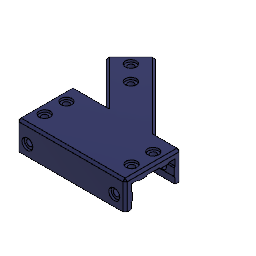
1-Side_Support_Top_Brace_Left v1 v1 (Autodesk Fusion 360 design; units mm, degrees)
Autodesk Fusion 360 part; units mm, degrees
mesh "Mesh1" [no effect]
sketch "Mesh Sectcion Sketch YZ" plane through (50, 0, 0) normal (1, 0, 0) x (0, 1, 0)
sketch "Sketch 2040" plane through (0, 0, 0) normal (1, 0, 0) x (0, 1, 0)
  line L0 (-4.607, 0) -> (-56.5, 0)
  line L1 (-56.5, 0.1599) -> (-56.5, 26.15)
  line L2 (-56.5, 26.15) -> (-50.75, 26.15)
  line L3 (-50.75, 26.15) -> (-50.75, 20.45)
  line L4 (-50.75, 20.45) -> (-49.75, 19.45)
  line L5 (-49.75, 19.45) -> (-49.75, 12.45)
  line L6 (-49.75, 12.45) -> (-50.75, 11.45)
  line L7 (-50.75, 11.45) -> (-50.75, 5.75)
  line L8 (-50.75, 5.75) -> (-45.05, 5.75)
  line L9 (-45.05, 5.75) -> (-44.05, 6.75)
  line L10 (-44.05, 6.75) -> (-37.05, 6.75)
  line L11 (-37.05, 6.75) -> (-36.05, 5.75)
  line L12 (-36.05, 5.75) -> (-25.05, 5.75)
  line L13 (-25.05, 5.75) -> (-24.05, 6.75)
  line L14 (-24.05, 6.75) -> (-17.05, 6.75)
  line L15 (-17.05, 6.75) -> (-16.05, 5.75)
  line L16 (-16.05, 5.75) -> (-10.35, 5.75)
  line L17 (-10.35, 5.75) -> (-10.35, 11.45)
  line L18 (-10.35, 11.45) -> (-11.35, 12.45)
  line L19 (-11.35, 12.45) -> (-11.35, 19.45)
  line L20 (-11.35, 19.45) -> (-10.35, 20.45)
  line L21 (-10.35, 20.45) -> (-10.35, 26.15)
  line L22 (-10.35, 26.15) -> (-4.6, 26.15)
  line L23 (-4.6, 26.15) -> (-4.6, 0.1599)
  line L24 (0, 0) -> (4.0383, 0) construction
  line L25 (-4.6, 0.1599) -> (-4.6, 0)
  line L26 (-4.607, 0) -> (-4.6, 0)
  line L27 (-56.5, 0.1599) -> (-56.5, 0)
  dimension "d2" = 135
  dimension "d3" = 135
  dimension "d4" = 135
  dimension "d5" = 135
  dimension "d6" = 135
  dimension "d7" = 135
  dimension "d8" = 135
  dimension "d9" = 135
  dimension "d10" = 135
  dimension "d13" = 7
  dimension "d14" = 7
  dimension "d15" = 7
  dimension "d16" = 7
  dimension "d18" = 5.75
  dimension "d23" = 26.15
  dimension "d25" = 5.75
  dimension "d27" = 1
  dimension "d28" = 5.7
  dimension "d31" = 4.6
  dimension "d33" = 51.9
  dimension "d34" = 40.4
  dimension "d35" = 5.8
  dimension "d36" = 5.7
  dimension "d37" = 5.7
  dimension "d38" = 5.7
  dimension "d39" = 5.7
  dimension "d40" = 11
  constraint perpendicular L0 L1
  constraint perpendicular L1 L2
  constraint perpendicular L2 L3
  constraint perpendicular L2 L5
  constraint perpendicular L2 L7
  constraint perpendicular L7 L8
  constraint perpendicular L7 L10
  constraint parallel L10 L12
  constraint parallel L12 L14
  constraint parallel L14 L16
  constraint perpendicular L16 L17
  constraint perpendicular L16 L19
  constraint perpendicular L21 L22
  constraint perpendicular L22 L23
  constraint equal L1 L23
  constraint equal L2 L22
  constraint equal L3 L21
  constraint equal L4 L20
  constraint equal L6 L18
  constraint equal L8 L16
  constraint equal L9 L13
  constraint equal L9 L11
  constraint equal L13 L15
  constraint equal L15 L18
  constraint equal L4 L6
  constraint coincident L24.start origin
  constraint horizontal L24
  constraint collinear L0 L24
  constraint collinear L2 L22
  constraint vertical L25
  constraint coincident L0 L25.end
  constraint perpendicular L25 L26
  constraint perpendicular L0 L27
  measures "d2" angle of L3 L4
  measures "d3" angle of L5 L6
  measures "d4" angle of L8 L9
  measures "d5" angle of L10 L11
  measures "d6" angle of L12 L13
  measures "d7" angle of L14 L15
  measures "d8" angle of L17 L18
  measures "d9" angle of L19 L20
  measures "d10" angle of L20 L21
  measures "d13" distance of L9.end L10.end
  measures "d14" distance of L13.end L14.end
  measures "d15" distance of L4.end L5.end
  measures "d16" distance of L18.end L19.end
  measures "d18" distance of L1.end L2.end
  measures "d23" distance of L0 L2
  measures "d25" distance of L0 L8
  measures "d27" distance of L3 L5
  measures "d28" distance of L2 L3.end
  measures "d31" distance of L24.start L23
  measures "d33" distance of L1 L23
  measures "d34" distance of L3 L21
  measures "d36" distance of L20.end L21.end
  measures "d37" distance of L16.end L17.end
  measures "d38" distance of L7.end L8.end
  measures "d39" distance of L15.end L16.end
  measures "d40" distance of L11.end L12.end
extrude "Extrude1" add sketch "Sketch 2040" along normal blind 54 and the other way blind 46 makes body 1
sketch "Mesh Section Sketch XY" plane through (0, 0, 3) normal (0, 0, 1) x (1, 0, 0)
sketch "Sketch 2040 Bottom holes" plane through (0, 0, 0) normal (0, 0, 1) x (1, 0, 0)
  line L0 (54, -24.05) -> (54, -17.05)
  line L1 (-46, -17.05) -> (-46, -24.05)
  line L2 (54, -44.05) -> (54, -37.05)
  line L3 (-46, -37.05) -> (-46, -44.05)
  line L4 (-46, -40.55) -> (54, -40.55) construction
  line L5 (-46, -20.55) -> (54, -20.55) construction
  line L6 (4, -20.55) -> (4, -40.55) construction
  line L7 (4, -30.55) -> (37.8098, -30.55) construction
  circle A0 centre (-36, -40.55) radius 2.75
  circle A1 centre (44, -40.55) radius 2.75
  circle A2 centre (-36, -20.55) radius 2.75
  circle A3 centre (44, -20.55) radius 2.75
  circle A4 centre (-36, -40.55) radius 5
  circle A5 centre (44, -40.55) radius 5
  circle A6 centre (-36, -20.55) radius 5
  circle A7 centre (44, -20.55) radius 5
  dimension "d45" = 5.5
  dimension "d46" = 10
  dimension "d49" = 2.25
  constraint midpoint L3 L4.start
  constraint midpoint L2 L4.end
  constraint midpoint L1 L5.start
  constraint midpoint L0 L5.end
  constraint midpoint L5 L6.start
  constraint midpoint L4 L6.end
  constraint midpoint L6 L7.start
  constraint perpendicular L6 L7
  constraint coincident L4 A0.centre
  constraint symmetric L6 A0 A1
  constraint symmetric L7 A0 A2
  constraint symmetric L7 A1 A3
  constraint symmetric L6 A4 A5
  constraint symmetric L7 A4 A6
  constraint symmetric L7 A5 A7
  measures "d45" diameter of A0
  measures "d46" distance of L3 A0.centre
extrude "Extrude3" cut sketch "Sketch 2040 Bottom holes" along normal blind 2 bodies 1
extrude "Extrude2" cut sketch "Sketch 2040 Bottom holes" along normal up to surface (6.75 mm away) contours A0 | A1 | A2 | A3 bodies 1
sketch "Sketch 2040 Side holes" plane through (0, 0, 0) normal (0, 1, 0) x (1, 0, 0)
  line L0 (54, -19.45) -> (54, -12.45)
  line L1 (-46, -12.45) -> (-46, -19.45)
  line L2 (-46, -15.95) -> (54, -15.95) construction
  circle A0 centre (-36, -15.95) radius 2.75
  circle A1 centre (-36, -15.95) radius 5
  line L3 (4, -15.95) -> (4, -28.2821) construction
  circle A2 centre (44, -15.95) radius 5
  circle A3 centre (44, -15.95) radius 2.75
  dimension "d52" = 5.5
  dimension "d53" = 10
  dimension "d54" = 2.25
  constraint midpoint L1 L2.start
  constraint midpoint L0 L2.end
  constraint coincident L2 A0.centre
  constraint midpoint L2 L3.start
  constraint perpendicular L2 L3
  constraint symmetric A0 L3 A3
  constraint symmetric A1 L3 A2
  measures "d52" diameter of A0
  measures "d53" distance of L1 A0.centre
extrude "Extrude4" cut sketch "Sketch 2040 Side holes" against normal through all contours A0 | A3 bodies 1
extrude "Extrude5" cut sketch "Sketch 2040 Side holes" against normal blind 2 from surface at -4.6 bodies 1
extrude "Extrude6" cut sketch "Sketch 2040 Side holes" along normal blind 2 from surface at -56.5 bodies 1
ref_plane "WorkPlane1" through (0, 0, 12.125) normal (-0.707107, 0.707107, 0) x (0, 0, 1)
sketch "Sketch6" plane through (-42.4264, 42.4264, 12.125) normal (-0.707107, 0.707107, 0) x (-0.707107, -0.707107, 0)
sketch "Sketch 2020" plane through (0, 0, 12.125) normal (-0.707107, 0.707107, 0) x (0, 0, 1)
  line L0 (-12.125, -35.7796) -> (-12.125, 34.9311)
  line L1 (14.025, -35.7796) -> (14.025, 34.9311)
  line L2 (14.025, 18) -> (-12.125, 18)
  line L3 (14.025, -14) -> (-12.125, -14)
  line L4 (-12.125, -3.2577) -> (-12.125, -39.9515)
  line L5 (8.325, 12.2) -> (7.325, 11.2)
  line L6 (8.325, 12.2) -> (9.7084, 12.2) construction
  line L7 (7.325, 11.2) -> (0.325, 11.2)
  line L8 (0.325, 11.2) -> (-0.675, 12.2)
  line L9 (-6.375, 6.5) -> (-5.375, 5.5)
  line L10 (-6.375, 6.5) -> (-4.9401, 6.5) construction
  line L11 (-0.675, -35.8857) -> (-6.375, -35.8857)
  line L12 (-5.375, 5.5) -> (-5.375, -1.5)
  line L13 (-5.375, -1.5) -> (-6.375, -2.5)
  line L14 (8.325, -8.2) -> (7.325, -7.2)
  line L15 (8.325, -8.2) -> (10.0345, -8.2) construction
  line L16 (7.325, -7.2) -> (0.325, -7.2)
  line L17 (0.325, -7.2) -> (-0.675, -8.2)
  line L18 (-6.375, -8.2) -> (-0.675, -8.2)
  line L19 (8.325, -8.2) -> (14.025, -8.2)
  line L20 (14.025, 12.2) -> (8.325, 12.2)
  line L21 (-0.675, 12.2) -> (-6.375, 12.2)
  line L22 (-6.375, 12.2) -> (-6.375, 6.5)
  line L23 (-6.375, -2.5) -> (-6.375, -8.2)
  point P0 (-12.125, 0)
  dimension "d67" = 135
  dimension "d68" = 135
  dimension "d69" = 1
  dimension "d70" = 45
  dimension "d71" = 135
  dimension "d72" = 1
  dimension "d73" = 135
  dimension "d74" = 135
  dimension "d75" = 1
  dimension "d76" = 7
  dimension "d81" = 7
  dimension "d83" = 32
  dimension "d84" = 14
  dimension "d90" = 20.4
  dimension "d91" = 20.4
  dimension "d92" = 5.8
  dimension "d93" = 5.9
  dimension "d95" = 5.75
  dimension "d96" = 5.7
  dimension "d97" = 5.7627
  dimension "d98" = 5.7
  dimension "d99" = 5.6
  constraint coincident L1 L2.start
  constraint coincident L0 L2.end
  constraint perpendicular L0 L2
  constraint coincident L1 L3.start
  constraint coincident L0 L3.end
  constraint perpendicular L0 L3
  constraint coincident L1 L20.start
  constraint perpendicular L1 L20
  constraint perpendicular L20 L22
  constraint coincident L1 L19.end
  constraint perpendicular L1 L18
  constraint horizontal L6
  constraint parallel L7 L20
  constraint horizontal L10
  constraint perpendicular L11 L12
  constraint horizontal L15
  constraint coincident L14.start L18
  constraint parallel L16 L18
  constraint collinear L18 L19
  constraint collinear L20 L21
  constraint collinear L22 L23
  constraint equal L7 L16
  constraint equal L7 L12
  constraint equal L19 L20
  measures "d67" angle of L5 L6
  measures "d68" angle of L7 L8
  measures "d69" distance of L7 L20
  measures "d70" angle of L9 L10
  measures "d71" angle of L12 L13
  measures "d72" distance of L12 L22
  measures "d73" angle of L14 L15
  measures "d74" angle of L16 L17
  measures "d75" distance of L16 L18
  measures "d76" distance of L5.end L7.end
  measures "d81" distance of L14.end L16.end
  measures "d83" distance of L2 L3
  measures "d84" distance of L3 P0
  measures "d90" distance of L1 L23
  measures "d91" distance of L19 L20
  measures "d92" distance of L2 L20
  measures "d95" distance of L2.end L22
  measures "d96" distance of L9.start L21
  measures "d98" distance of L8.end L22
extrude "Extrude7" add sketch "Sketch 2020" along normal blind 61.5 from surface at 1.9 contours L0 L1 L2 L3 L4 L5 L7 L8 L9 L12 L13 L14 L16 L17 L18 L19 L20 L21 L22 L23 bodies 1
extrude "Extrude8" add sketch "Sketch 2020" along normal up to surface (1.9 mm away) bodies 1
move_face "OffsetFaces1" offset 25 1 faces at (1.176, 1.176, 17.4333) on bodies 1
sketch "Sketch 2020 Bottom holes" plane through (0, 0, 6.75) normal (0, 0, 1) x (-1, 0, 0)
  line L0 (45.8912, -43.7699) -> (40.9415, -48.7197)
  line L1 (43.4164, -46.2448) -> (36.3453, -39.1737) construction
  line L2 (43.4164, -46.2448) -> (53.4164, -46.2448) construction
  circle A0 centre (36.3453, -39.1737) radius 2.75
  circle A1 centre (36.3453, -39.1737) radius 5
  circle A2 centre (22.2032, -25.0316) radius 5
  circle A3 centre (22.2032, -25.0316) radius 2.75
  dimension "d106" = 135
  dimension "d107" = 10
  dimension "d108" = 5.5
  dimension "d109" = 2.25
  dimension "d112" = 20
  dimension "d113" = 0
  constraint horizontal L2
  constraint midpoint L0 L1.start
  constraint coincident L1.end A0.centre
  measures "d106" angle of L1 L2
  measures "d107" distance of L1.start L1.end
  measures "d108" diameter of A0
extrude "Extrude9" cut sketch "Sketch 2020 Bottom holes" against normal up to surface (6.75 mm away) contours A0 | A3 bodies 1
extrude "Extrude10" cut sketch "Sketch 2020 Bottom holes" along normal blind 2 from surface at -6.75 bodies 1
sketch "Sketch 2020 side holes" plane through (7.9196, 7.9196, 0) normal (-0.707107, -0.707107, 0) x (0.707107, -0.707107, 0)
  line L0 (-63.4, 12.45) -> (-63.4, 19.45)
  line L1 (-63.4, 15.95) -> (-53.4, 15.95) construction
  circle A0 centre (-53.4, 15.95) radius 2.75
  circle A1 centre (-53.4, 15.95) radius 5
  circle A2 centre (-33.4, 15.95) radius 5
  circle A3 centre (-33.4, 15.95) radius 2.75
  dimension "d119" = 10
  dimension "d120" = 5.5
  dimension "d121" = 2.25
  dimension "d124" = 20
  dimension "d125" = 0
  constraint midpoint L0 L1.start
  constraint perpendicular L0 L1
  constraint coincident L1.end A0.centre
  measures "d119" distance of L1.start L1.end
  measures "d120" diameter of A0
extrude "Extrude11" cut sketch "Sketch 2020 side holes" along normal through all and the other way through all contours A0 | A3 bodies 1
extrude "Extrude12" cut sketch "Sketch 2020 side holes" along normal blind 2 from surface at -6.8 bodies 1
extrude "Extrude13" cut sketch "Sketch 2020 side holes" against normal blind 2 from surface at 25.2 bodies 1
extrude "Extrude14" add 1 faces at (-12.6667, -50.75, 24.25) along direction (0, 1, 0) blind 0.1 on bodies 1 bodies 1
extrude "Extrude15" add 1 faces at (-12.6667, -50.75, 9.55) along direction (0, 1, 0) blind 0.1 on bodies 1 bodies 1
extrude "Extrude16" add 1 faces at (20.6667, -10.35, 22.35) along direction (0, -1, 0) blind 0.1 on bodies 1 bodies 1
extrude "Extrude17" add 1 faces at (20.6667, -10.35, 7.65) along direction (0, -1, 0) blind 0.1 on bodies 1 bodies 1
delete_face "DeleteFace1" 1 faces at (20.6667, -10.3833, 11.45) on bodies 1
delete_face "DeleteFace2" 1 faces at (20.6667, -10.3833, 20.45) on bodies 1
delete_face "DeleteFace3" 1 faces at (20.6667, -50.7167, 20.45) on bodies 1
delete_face "DeleteFace4" 1 faces at (20.6667, -50.7167, 11.45) on bodies 1
chamfer "Chamfer1" distance 2 angle 45 14 edges at (-1.0234, 26.4792, 0) (42.0279, -4.6, 0) (54, -30.55, 0) (4, -56.5, 0) (-46, -30.55, 0) (-30.5995, -4.6, 0) (-43.4164, 46.2448, 0) (54, -56.5, 13.075) (54, -4.6, 13.075) (-32.1026, 57.5585, 13.075) (-54.7301, 34.9311, 13.075) (-46, -4.6, 13.075) (-46, -56.5, 13.075) (-34.9645, 15.1655, 0) on bodies 1
mirror "Mirror1" about plane through (0, -4.607, 0) normal (0, 0, -1) of bodies 1 makes body 2
delete_body "RemoveBody1" bodies 1
equation "d14 = d13"
equation "d15 = d13"
equation "d16 = d13"
equation "d25 = d18"
equation "d38 = d28"
equation "d72 = d69"
equation "d75 = d69"
equation "d98 = d96"
